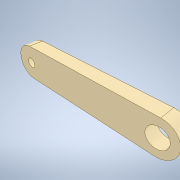
# Autodesk Inventor part: Рычаг натяжителя
Saved by Autodesk Inventor 2021.1 (Build 251245010, 245A)
## iProperties
Created: 2026-04-14
Part Number: Рычаг натяжителя
Material: Типовые
Document SubType Name: Modeling
Designer: Андрей Тарасов
Density: 1 g/cm^3
Appearance: По умолчанию
Author: Андрей Тарасов
Autodesk Inventor part; units mm, degrees
ref_plane "YZ Plane" through (0, 0, 0) normal (1, 0, 0) x (0, 1, 0)
ref_plane "XZ Plane" through (0, 0, 0) normal (0, 1, 0) x (-1, 0, 0)
ref_plane "XY Plane" through (0, 0, 0) normal (0, 0, 1) x (1, 0, 0)
sketch "Эскиз1" plane through (0, 0, 0) normal (0, 0, 1) x (1, 0, 0)
  line L0 (0, 0) -> (57, 0) construction
  line L1 (0, -7) -> (57, -7)
  line L2 (57, 7) -> (0, 7)
  arc A0 (0, 7) -> (0, -7) centre (0, 0) ccw
  arc A1 (57, -7) -> (57, 7) centre (57, 0) ccw
  circle A2 centre (57, 0) radius 4
  circle A3 centre (0, 0) radius 2
  point P0 (28.5, 0)
  dimension "d0" = 8
  dimension "d1" = 4
  dimension "d2" = 57
  dimension "d3" = 7
  constraints: 8 end point, 4 centre point, 4 point on circle, 4 tangent, 2 coincident, 1 horizontal, 1 midpoint, 1 parallel
  measures "d0" diameter of A2
  measures "d1" diameter of A3
  measures "d2" distance of L0.start L0.end
  measures "d3" radius of A1
extrude "Выдавливание1" add sketch "Эскиз1" along normal blind 6
